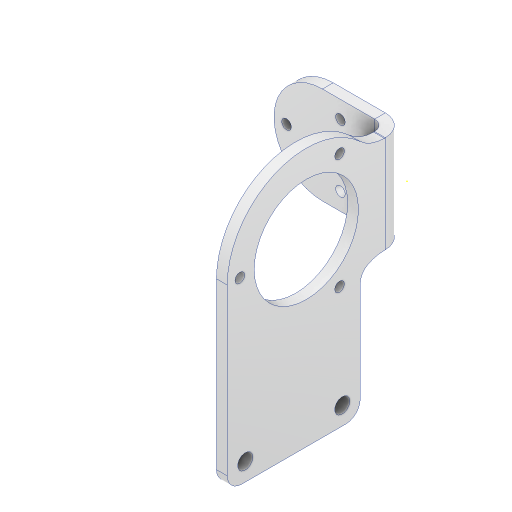
# Autodesk Inventor part: hand_plate
Saved by Autodesk Inventor 2024.3 (Build 283343000, 343)
## iProperties
Created: 2024-10-15
Part Number: hand_plate
Material: アルミニウム 6061
Document SubType Name: Sheet Metal
Designer: haya
Density: 2.7 g/cm^3
Sheet Metal Rule: Default_mm
Appearance: アルミニウム - フラット
Mass: 16.4969 g
Surface Area: 52.5071 cm^2
Volume: 6.10997 cm^3
Author: haya
Autodesk Inventor part; units mm, degrees
note: some values were not read from the file. Chosen so that the rebuilt part matches the saved one: direction of "穴1"; direction of "穴2"; flange form of "プレート2"; direction of "穴3".
ref_plane "YZ Plane" through (0, 0, 0) normal (1, 0, 0) x (0, 1, 0)
ref_plane "XZ Plane" through (0, 0, 0) normal (0, 1, 0) x (-1, 0, 0)
ref_plane "XY Plane" through (0, 0, 0) normal (0, 0, 1) x (1, 0, 0)
sketch "スケッチ1" plane through (0, 0, 0) normal (0, 0, 1) x (1, 0, 0)
  circle A0 centre (0, 0) radius 13.5
  line L0 (0, 13.5) -> (14.5, 13.5)
  line L1 (14.5, 13.5) -> (14.5, -13.5)
  line L2 (14.5, -13.5) -> (0, -13.5)
  line L3 (0, -13.5) -> (0, 13.5)
  line L4 (0, 0) -> (14.5, 0) construction
  point P0 (0, 13.5)
  point P1 (0, -13.5)
  point P2 (0, -13.5)
  dimension "d0" = 27
  dimension "d1" = 27
  dimension "d2" = 14.5
  measures "d0" diameter of A0
  measures "d1" distance of L2.end L0.start
  measures "d2" distance of L1.end L2.end
extrude "プレート1" add sketch "スケッチ1" along normal blind 3
sketch "スケッチ2" plane through (17.5, 13.5, 6) normal (1, 0, 0) x (0, 1, 0)
  line L0 (-27, 0) -> (0, 0)
  line L1 (0, 0) -> (0, 19)
  line L2 (0, 19) -> (-27, 19)
  line L3 (-27, 19) -> (-27, 0)
  constraints: 6 end point, 1 horizontal, 1 perpendicular, 1 vertical
edge flange "フランジ1" height 25 angle 90 thickness 3 bend radius 3 thickness toward (1, 0, 0) relief tear relief width 3 relief depth 1.5 edges at (14.5, 0, 3) wall of the first edge with corners at (17.5, -13.5, 6) (17.5, 13.5, 6) (17.5, 13.5, 25) (17.5, -13.5, 25)
bend "曲げ1"
corner "コーナー1"
sketch "スケッチ3" plane through (0, 0, 0) normal (0, 0, -1) x (-1, 0, 0)
  point P0 (0, 0)
  point P1 (10, 0)
  point P2 (-5, 8.6603)
  point P3 (-5, -8.6603)
  dimension "d14" = 10
  dimension "d17" = 360
  constraints: 4 other
  measures "d14" distance of point (10, 0) point (0, 0)
hole "穴1" at (-10, 0, 0) at (5, 8.6603, 0) at (5, -8.6603, 0) direction (0, 0, 1) diameter 2.7 depth 3
sketch "スケッチ4" plane through (20.5, -13.5, 25) normal (1, 0, 0) x (0, 0, -1)
  circle A0 centre (-3, 13.5) radius 22
  line L0 (25, 27) -> (25, 0) projected
  line L1 (0, 27) -> (19, 27) projected
  point P0 (25, 13.5)
  dimension "d26" = 44
  dimension "d29" = 28
  dimension "d62" = 13.5
  constraints: 1 centre point
  measures "d26" diameter of A0
  measures "d29" distance from line of A0.centre L0
  measures "d62" distance from line of A0.centre L1
extrude "押し出し1" add sketch "スケッチ4" against normal up to surface (3 mm away)
sketch "スケッチ5" plane through (20.5, -13.5, 6) normal (1, 0, 0) x (0, 0, -1)
  arc A0 (-4.629, 27) -> (-4.629, 0) centre (-22, 13.5) ccw projected
  circle A1 centre (-22, 13.5) radius 14.5
  point P0 (6, 13.5)
  dimension "d30" = 29
  constraints: 1 centre point, 1 coincident
  measures "d30" diameter of A1
extrude "押し出し2" cut sketch "スケッチ5" against normal up to surface (3 mm away)
sketch "スケッチ6" plane through (20.5, 0, 28) normal (1, 0, 0) x (0, 0, 1)
  point P0 (-28, 0)
sketch "スケッチ7" plane through (20.5, -13.5, 6) normal (1, 0, 0) x (0, 0, -1)
  circle A0 centre (-22, 13.5) radius 14.5 projected
  point P0 (6, 13.5)
  point P1 (-40.5, 13.5)
  point P2 (-12.75, -2.5215)
  point P3 (-12.75, 29.5215)
  dimension "d33" = 18.5
  dimension "d36" = 360
  constraints: 4 other
  measures "d33" distance of point (-40.5, 13.5) A0.centre
hole "穴2" at (20.5, 0, 46.5) at (20.5, -16.0215, 18.75) at (20.5, 16.0215, 18.75) direction (-1, 0, 0) diameter 2.7 depth 3
fillet "フィレット1" radius 10 2 edges at (19, 13.5, 10.629) (19, -13.5, 10.629)
sketch "スケッチ8" plane through (20.5, -13.5, 6) normal (1, 0, 0) x (0, 0, -1)
  arc A0 (-7.0676, 29.6563) -> (-7.0676, -2.6562) centre (-22, 13.5) ccw projected
  line L0 (-44, 13.5) -> (-7, 13.5)
  line L1 (-7, 13.5) -> (-7, -36.5)
  line L2 (-7, -36.5) -> (-44, -36.5)
  line L3 (-44, -36.5) -> (-44, 13.5)
  arc A1 (-7.0676, 29.6562) -> (-0.2802, 27) centre (-0.2802, 37) ccw projected
  line L4 (0, 0) -> (0, 27) projected
  line L5 (0, 0) -> (-0.2802, 0) projected
  arc A2 (-0.2802, 0) -> (-7.0676, -2.6562) centre (-0.2802, -10) ccw projected
  arc A3 (-7.0676, 29.6562) -> (-7.0676, -2.6562) centre (-22, 13.5) ccw projected
  circle A4 centre (-12.75, 29.5215) radius 1.35 projected
  circle A5 centre (-12.75, -2.5215) radius 1.35 projected
  circle A6 centre (-22, 13.5) radius 14.5 projected
  circle A7 centre (-40.5, 13.5) radius 1.35 projected
  point P0 (6, 13.5)
  point P1 (-11.4, 29.5215)
  point P2 (-11.4, 29.5215)
  point P3 (-11.4, -2.5215)
  point P4 (-11.4, -2.5215)
  point P5 (-7.5, 13.5)
  point P6 (-7.5, 13.5)
  point P7 (-39.15, 13.5)
  point P8 (-39.15, 13.5)
  point P9 (-7, -2.5943)
  point P10 (-7.0676, -2.6562)
  dimension "d46" = 50
  dimension "d47" = 37
  constraints: 8 end point, 2 parallel, 1 horizontal, 1 perpendicular, 1 point on circle
  measures "d46" distance of L2.end L0.start
  measures "d47" distance of L1.end L2.end
extrude "押し出し3" add sketch "スケッチ8" against normal up to surface (3 mm away) contours A0 A2 L1 L2 L3
fillet "フィレット2" radius 4 1 edges at (19, -16.0943, 13)
fillet "フィレット3" radius 4 2 edges at (19, -50, 13) (19, -50, 50)
sketch "スケッチ9" plane through (20.5, -13.5, 6) normal (1, 0, 0) x (0, 0, -1)
  line L0 (-44, 13.5) -> (-44, -32.5) projected
  line L1 (-44, -31.5) -> (-6.9219, -31.5) construction
  line L2 (-40, -36.5) -> (-11, -36.5) projected
  line L3 (-7, -32.5) -> (-7, -4.6519) projected
  point P0 (6, 13.5)
  point P1 (-39, -31.5)
  point P2 (-12, -31.5)
  dimension "d52" = 5
  dimension "d53" = 5
  dimension "d54" = 5
  constraints: 3 point on line, 2 end point, 1 horizontal
  measures "d52" distance between parallel lines of L1 L2
  measures "d53" distance from line of point (-12, -31.5) L3
  measures "d54" distance from line of point (-39, -31.5) L0
hole "穴3" at (20.5, -45, 45) at (20.5, -45, 18) direction (-1, 0, 0) diameter 4.2 depth 3
equation "\"d24\" = Thickness"
equation "\"d60\" = Thickness"
equation "\"d3\" = Thickness"
equation "\"d4\" = BendReliefWidth"
equation "\"d5\" = BendReliefDepth"
equation "\"d6\" = MinimumRemnant"
equation "\"d7\" = TransitionRadius"
equation "\"d10\" = BendRadius"
equation "\"d11\" = CornerReliefSize"
equation "\"d12\" = GapSize"
equation "\"d13\" = JacobiRadiusSize"
equation "\"BendRadius\" = Thickness"
equation "\"BendReliefWidth\" = Thickness"
equation "\"BendReliefDepth\" = 0.5 * Thickness"
equation "\"CornerReliefSize\" = 4 * Thickness"
equation "\"MinimumRemnant\" = 2 * Thickness"
equation "\"TransitionRadius\" = BendRadius"
equation "\"JacobiRadiusSize\" = BendRadius"
equation "\"GapSize\" = Thickness"
equation "\"Thickness\" = 3"
